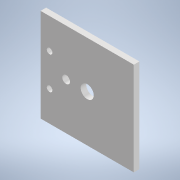
# Autodesk Inventor part: arm2
Saved by Autodesk Inventor 2021 (Build 250183000, 183)
## iProperties
Created: 2022-05-25
Part Number: arm2
Material: Generic
Document SubType Name: Modeling
Designer: techv
Density: 1 g/cm^3
Appearance: Default
Author: techv
Autodesk Inventor part; units mm, degrees
ref_plane "YZ Plane" through (0, 0, 0) normal (1, 0, 0) x (0, 1, 0)
ref_plane "XZ Plane" through (0, 0, 0) normal (0, 1, 0) x (-1, 0, 0)
ref_plane "XY Plane" through (0, 0, 0) normal (0, 0, 1) x (1, 0, 0)
sketch "Sketch1" plane through (0, 0, 0) normal (0, 0, 1) x (1, 0, 0)
  ellipse E0 centre (0, 0) end of major axis (0, 3.5) minor radius 3.5 projected
  arc A0 (-2.0076, 1.85) -> (-2.0076, -1.85) centre (0, 0) ccw projected
  line L0 (-2.0076, 1.85) -> (2.0076, 1.85) projected
  arc A1 (2.0076, -1.85) -> (2.0076, 1.85) centre (0, 0) ccw projected
  line L1 (2.0076, -1.85) -> (-2.0076, -1.85) projected
  line L2 (-50, -25) -> (50, -25)
  line L3 (50, -25) -> (50, 25)
  line L4 (50, 25) -> (-50, 25)
  line L5 (-50, 25) -> (-50, -25)
  line L6 (-50, -25) -> (50, 25) construction
  line L7 (50, -25) -> (-50, 25) construction
  line L8 (-25, -25) -> (-25, 25)
  line L9 (25, -25) -> (25, 25)
  circle A2 centre (0, 0) radius 6.15
  point P0 (0, 0)
  dimension "d0" = 100
  dimension "d1" = 50
  dimension "d4" = 25
  dimension "d5" = 50
  dimension "d10" = 12.3
  constraints: 16 end point, 4 point on line, 3 perpendicular, 2 midpoint, 2 parallel, 1 centre point, 1 coincident, 1 horizontal, 1 other
  measures "d0" distance of L4.end L3.end
  measures "d1" distance of L3.end L2.end
  measures "d4" distance between parallel lines of L3 L9
  measures "d5" distance between parallel lines of L8 L9
  measures "d10" diameter of A2
extrude "Extrusion1" add sketch "Sketch1" against normal blind 3 contours L8 L4 L9 L2
sketch "Sketch2" plane through (0, 0, -3) normal (0, 0, -1) x (-1, 0, 0)
  circle A0 centre (20.11, -8.75) radius 1.5 projected
  circle A1 centre (11.22, 0) radius 2.08 projected
  circle A2 centre (20.11, 8.75) radius 1.5 projected
  point P0 (0, 0)
extrude "Extrusion2" cut sketch "Sketch2" against normal through all
sketch "Sketch3" plane through (-25, -25, 0) normal (-1, 0, 0) x (0, 0, 1)
  line L0 (0, 50) -> (0, 0) projected
  line L1 (0, 50) -> (-3, 50) projected
  line L2 (-3, 0) -> (-3, 50) projected
  line L3 (0, 0) -> (-3, 0) projected
  point P0 (0, 25)
extrude "Extrusion3" add sketch "Sketch3" along normal blind 10
sketch "Sketch4" plane through (0, 0, -3) normal (0, 0, -1) x (-1, 0, 0)
  circle A0 centre (20.11, -8.75) radius 1.5 projected
  circle A1 centre (20.11, 8.75) radius 1.5 projected
  point P0 (0, 0)
extrude "Extrusion4" cut sketch "Sketch4" against normal through all
body "Solid1"
